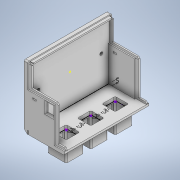
# Autodesk Inventor part: sUPORTE
Saved by Autodesk Inventor 2022 (Build 260153000, 153)
## iProperties
Created: 2022-12-13
Part Number: sUPORTE
Material: Genérico
Document SubType Name: Modeling
Designer: gugarauj07
Density: 1 g/cm^3
Appearance: Padrão
Author: gugarauj07
Autodesk Inventor part; units mm, degrees
ref_plane "YZ Plane" through (0, 0, 0) normal (1, 0, 0) x (0, 1, 0)
ref_plane "XZ Plane" through (0, 0, 0) normal (0, 1, 0) x (-1, 0, 0)
ref_plane "XY Plane" through (0, 0, 0) normal (0, 0, 1) x (1, 0, 0)
sketch "Esboço1" plane through (0, 0, 0) normal (1, 0, 0) x (0, 1, 0)
  line L0 (40.5, 60) -> (-42.5, 60)
  line L1 (-42.5, 60) -> (-42.5, -60)
  line L2 (-42.5, -60) -> (40.5, -60)
  line L3 (42.5, -58) -> (42.5, 58)
  line L4 (-42.5, 60) -> (42.5, -60) construction
  arc A0 (42.5, 58) -> (40.5, 60) centre (40.5, 58) ccw
  arc A1 (40.5, -60) -> (42.5, -58) centre (40.5, -58) ccw
  point P0 (0, 0)
  dimension "d0" = 85
  dimension "d1" = 120
  dimension "d4" = 2
  constraints: 10 end point, 4 point on circle, 4 tangent, 2 centre point, 2 parallel, 2 point on line, 1 equal radius, 1 horizontal, 1 midpoint, 1 perpendicular
  measures "d0" distance of L4.end L1.end
  measures "d1" distance of L0.end L1.end
  measures "d4" radius of A0
extrude "Extrusão1" add sketch "Esboço1" along normal blind 5
sketch "Esboço4" plane through (5, 0, 0) normal (1, 0, 0) x (0, 0, -1)
  line L0 (-60, -42.5) -> (60, -42.5) projected
  line L1 (-60, -42.5) -> (60, -42.5)
  line L2 (60, -42.5) -> (60, -47.5)
  line L3 (60, -47.5) -> (-60, -47.5)
  line L4 (-60, -47.5) -> (-60, -42.5)
  point P0 (0, 0)
  point P1 (60, -42.5)
  dimension "d33" = 5
  constraints: 8 end point, 2 parallel, 1 horizontal, 1 perpendicular
  measures "d33" distance of L1.end L2.end
extrude "Extrusão3" add sketch "Esboço4" against normal blind 5
sketch "Esboço5" plane through (5, 0, 0) normal (1, 0, 0) x (0, 0, -1)
  line L0 (-60, 40.5) -> (-60, -47.5) projected
  line L1 (60, 40.5) -> (60, -47.5) projected
  line L2 (-60, -47.5) -> (60, -47.5)
  line L3 (60, -47.5) -> (60, -42.5)
  line L4 (60, -42.5) -> (-60, -42.5)
  line L5 (-60, -42.5) -> (-60, -47.5)
  point P0 (0, 0)
  point P1 (60, -47.5)
  dimension "d36" = 5
  constraints: 8 end point, 2 parallel, 1 horizontal, 1 perpendicular, 1 point on line
  measures "d36" distance of L3.end L2.end
extrude "Extrusão4" add sketch "Esboço5" along normal blind 53.158
chamfer "Chanfro2" distance 4 angle 45 1 edges at (0, -47.5, 0)
chamfer "Chanfro3" distance 2 angle 45 1 edges at (58.158, -47.5, 0)
sketch "Esboço7" plane through (5, 0, 0) normal (1, 0, 0) x (0, 0, -1)
  circle A0 centre (-45, 0) radius 3
  circle A1 centre (45, 0) radius 3
  point P0 (0, 0)
  dimension "d61" = 6
  dimension "d62" = 6
  constraints: 2 centre point
  measures "d61" diameter of A0
  measures "d62" diameter of A1
hole "Furo3" at (5, 0, 45) direction (-1, 0, 0) diameter 4.3434 depth 16.265 tip angle 118 thread size "12-24 UNC" class "2B" standard "ANSI Unified Screw Threads"
hole "Furo4" at (5, 0, -45) direction (-1, 0, 0) diameter 4.3434 depth 16.265 tip angle 118 thread size "12-24 UNC" class "2B" standard "ANSI Unified Screw Threads"
sketch "Esboço9" plane through (4, -47.5, -60) normal (0, -1, 0) x (1, 0, 0)
  line L0 (40.5, 87.5) -> (40.5, 102.5) projected
  line L1 (23.5, 85.5) -> (38.5, 85.5) projected
  line L2 (38.5, 104.5) -> (23.5, 104.5) projected
  line L3 (21.5, 102.5) -> (21.5, 87.5) projected
  line L4 (23.5, 15.5) -> (38.5, 15.5) projected
  line L5 (43.5, 12.5) -> (31, 12.5)
  line L6 (31, 12.5) -> (16.5, 12.5)
  line L7 (16.5, 95) -> (16.5, 107.5)
  line L8 (16.5, 107.5) -> (43.5, 107.5)
  line L9 (43.5, 107.5) -> (43.5, 95)
  line L10 (38.5, 34.5) -> (23.5, 34.5) projected
  line L11 (31, 34.5) -> (31, 37.5)
  line L12 (23.5, 50.5) -> (38.5, 50.5) projected
  line L13 (31, 50.5) -> (31, 47.5)
  line L14 (38.5, 69.5) -> (23.5, 69.5) projected
  line L15 (31, 69.5) -> (31, 72.5)
  line L16 (31, 85.5) -> (31, 82.5)
  line L17 (43.5, 82.5) -> (16.5, 82.5)
  line L18 (43.5, 72.5) -> (16.5, 72.5)
  line L19 (43.5, 47.5) -> (16.5, 47.5)
  line L20 (43.5, 37.5) -> (16.5, 37.5)
  line L21 (43.5, 95) -> (43.5, 82.5)
  line L22 (16.5, 82.5) -> (16.5, 95)
  line L23 (16.5, 12.5) -> (16.5, 37.5)
  line L24 (16.5, 47.5) -> (16.5, 72.5)
  line L25 (43.5, 72.5) -> (43.5, 47.5)
  line L26 (43.5, 37.5) -> (43.5, 12.5)
  line L27 (31, 104.5) -> (31, 107.5)
  line L28 (31, 15.5) -> (31, 12.5)
  arc A0 (23.5, 104.5) -> (21.5, 102.5) centre (23.5, 102.5) ccw projected
  arc A1 (23.5, 104.5) -> (21.5, 102.5) centre (23.5, 102.5) ccw
  arc A2 (40.5, 102.5) -> (38.5, 104.5) centre (38.5, 102.5) ccw
  arc A3 (38.5, 85.5) -> (40.5, 87.5) centre (38.5, 87.5) ccw projected
  arc A4 (38.5, 85.5) -> (40.5, 87.5) centre (38.5, 87.5) ccw
  arc A5 (21.5, 87.5) -> (23.5, 85.5) centre (23.5, 87.5) ccw projected
  arc A6 (21.5, 87.5) -> (23.5, 85.5) centre (23.5, 87.5) ccw
  line L29 (21.5, 102.5) -> (21.5, 87.5)
  line L30 (23.5, 104.5) -> (31, 104.5)
  line L31 (31, 104.5) -> (38.5, 104.5)
  arc A7 (40.5, 102.5) -> (38.5, 104.5) centre (38.5, 102.5) ccw projected
  line L32 (40.5, 102.5) -> (40.5, 87.5)
  line L33 (38.5, 85.5) -> (31, 85.5)
  line L34 (23.5, 85.5) -> (31, 85.5)
  line L35 (31, 69.5) -> (29.1751, 69.5)
  arc A8 (23.5, 69.5) -> (21.5, 67.5) centre (23.5, 67.5) ccw projected
  line L36 (31, 69.5) -> (23.5, 69.5)
  line L37 (21.5, 67.5) -> (21.5, 52.5) projected
  line L38 (21.5, 67.5) -> (21.5, 52.5)
  arc A9 (21.5, 52.5) -> (23.5, 50.5) centre (23.5, 52.5) ccw projected
  line L39 (23.5, 50.5) -> (31, 50.5)
  line L40 (31, 50.5) -> (38.5, 50.5)
  arc A10 (38.5, 50.5) -> (40.5, 52.5) centre (38.5, 52.5) ccw projected
  line L41 (40.5, 52.5) -> (40.5, 67.5)
  line L42 (38.5, 69.5) -> (31, 69.5)
  line L43 (31, 34.5) -> (38.5, 34.5)
  arc A11 (40.5, 32.5) -> (38.5, 34.5) centre (38.5, 32.5) ccw projected
  arc A12 (38.5, 15.5) -> (40.5, 17.5) centre (38.5, 17.5) ccw projected
  line L44 (40.5, 32.5) -> (40.5, 17.5)
  line L45 (38.5, 15.5) -> (31, 15.5)
  arc A13 (21.5, 17.5) -> (23.5, 15.5) centre (23.5, 17.5) ccw projected
  line L46 (31, 15.5) -> (23.5, 15.5)
  line L47 (21.5, 32.5) -> (21.5, 17.5) projected
  line L48 (21.5, 17.5) -> (21.5, 32.5)
  line L49 (23.5, 34.5) -> (31, 34.5)
  arc A14 (23.5, 34.5) -> (21.5, 32.5) centre (23.5, 32.5) ccw projected
  arc A15 (23.5, 34.5) -> (21.5, 32.5) centre (23.5, 32.5) ccw
  arc A16 (21.5, 17.5) -> (23.5, 15.5) centre (23.5, 17.5) ccw
  arc A17 (38.5, 15.5) -> (40.5, 17.5) centre (38.5, 17.5) ccw
  arc A18 (40.5, 32.5) -> (38.5, 34.5) centre (38.5, 32.5) ccw
  arc A19 (38.5, 50.5) -> (40.5, 52.5) centre (38.5, 52.5) ccw
  arc A20 (21.5, 52.5) -> (23.5, 50.5) centre (23.5, 52.5) ccw
  arc A21 (23.5, 69.5) -> (21.5, 67.5) centre (23.5, 67.5) ccw
  arc A22 (40.5, 67.5) -> (38.5, 69.5) centre (38.5, 67.5) ccw projected
  arc A23 (40.5, 67.5) -> (38.5, 69.5) centre (38.5, 67.5) ccw
  point P0 (-4, 60)
  dimension "d102" = 3
  dimension "d103" = 3
  dimension "d104" = 3
  dimension "d105" = 3
  constraints: 80 end point, 25 point on circle, 21 perpendicular, 14 collinear, 12 centre point, 11 tangent, 10 vertical, 6 midpoint, 3 point on line, 2 horizontal, 1 concentric
  measures "d102" distance of L11.start L11.end
  measures "d103" distance of L13.start L13.end
  measures "d104" distance of L15.start L15.end
  measures "d105" distance of L16.start L16.end
extrude "Extrusão7" add sketch "Esboço9" along normal blind 21 contours L16 L17 L22 L7 L8 L27 L2 A0 L3 A5 L1 | L4 L28 L6 L23 L20 L11 L10 A14 L47 A13 | L12 L13 L19 L24 L18 L15 L14 A8 L37 A9
extrude "Extrusão9" add sketch "Esboço9" along normal blind 21 contours L0 A2 L2 L27 L8 L9 L21 L17 L16 L1 A3 | L4 A12 L44 A11 L10 L11 L20 L26 L5 L28 | L12 A10 L41 A22 L14 L15 L18 L25 L19 L13
fillet "Arredondamento1" radius 2 12 edges at (47.5, -58, -47.5) (20.5, -58, -47.5) (20.5, -58, -22.5) (47.5, -58, -22.5) (47.5, -58, -12.5) (20.5, -58, -12.5) (20.5, -58, 12.5) (47.5, -58, 12.5) (47.5, -58, 22.5) (20.5, -58, 22.5) (20.5, -58, 47.5) (47.5, -58, 47.5)
sketch "Esboço12" plane through (5, 0, 0) normal (1, 0, 0) x (0, 0, -1)
  line L0 (60, -42.5) -> (60, 40.5) projected
  line L1 (60, -42.5) -> (55, -42.5)
  line L2 (55, -42.5) -> (55, 7.5)
  line L3 (55, 7.5) -> (60, 7.5)
  line L4 (60, 7.5) -> (60, -42.5)
  line L5 (60, -42.5) -> (-60, -42.5) projected
  line L6 (-60, -42.5) -> (-55, -42.5)
  line L7 (-55, -42.5) -> (-55, 7.5)
  line L8 (-55, 7.5) -> (-60, 7.5)
  line L9 (-60, 7.5) -> (-60, -42.5)
  point P0 (0, 0)
  dimension "d123" = 5
  dimension "d124" = 50
  dimension "d125" = 5
  dimension "d126" = 50
  constraints: 16 end point, 4 parallel, 2 horizontal, 2 perpendicular
  measures "d123" distance of L2.end L3.end
  measures "d124" distance of L1.end L2.end
  measures "d125" distance of L8.end L7.end
  measures "d126" distance of L7.end L6.end
extrude "Extrusão10" add sketch "Esboço12" along normal blind 38
sketch "Esboço13" plane through (43, 0, 0) normal (1, 0, 0) x (0, 0, -1)
  line L0 (-60, 40.5) -> (-60, -43.5) projected
  line L1 (-60, -42.5141) -> (-58.5, -42.5141)
  line L2 (-60, -42.5141) -> (-58.5, -42.5141) construction
  line L3 (60, -42.5) -> (-60, -42.5) projected
  line L4 (-55, 7.5) -> (-60, 7.5) projected
  line L5 (-58.5, -42.5) -> (-56.5, -42.5)
  line L6 (-56.5, -42.5) -> (-56.5, 7.5)
  line L7 (-56.5, 7.5) -> (-58.5, 7.5)
  line L8 (-58.5, 7.5) -> (-58.5, -42.5)
  line L9 (58, 42.5) -> (-58, 42.5) projected
  line L10 (-57.5, 42.5) -> (-56, 42.5) construction
  line L11 (-58.5, 7.5) -> (-56.5, 7.5)
  line L12 (60, -42.5) -> (55, -42.5) projected
  line L13 (60, -42.5) -> (58.5, -42.5)
  line L14 (55, 7.5) -> (60, 7.5) projected
  line L15 (58.5, -42.5) -> (56.5, -42.5)
  line L16 (56.5, -42.5) -> (56.5, 7.5)
  line L17 (56.5, 7.5) -> (58.5, 7.5)
  line L18 (58.5, 7.5) -> (58.5, -42.5)
  point P0 (0, 0)
  dimension "d129" = 1.5
  dimension "d130" = 0
  dimension "d135" = 1.5
  dimension "d136" = 2
  constraints: 26 end point, 6 point on line, 5 horizontal, 4 parallel, 3 perpendicular, 1 collinear
  measures "d129" distance of L1.start L1.end
  measures "d130" distance between parallel lines of L1 L2
  measures "d135" distance of L3.start L13.end
  measures "d136" distance of L16.end L17.end
extrude "Extrusão11" add sketch "Esboço13" along normal blind 4 contours L4 L6 L3 L8 | L3 L16 L14 L18
extrude "Extrusão12" cut sketch "Esboço9" against normal blind 6 contours A3 L1 A5 L3 A0 L2 A2 L0 | A13 L47 A14 L10 A11 L44 A12 L4 | A9 L37 A8 L14 A22 L41 A10 L12
sketch "Esboço14" plane through (5, 0, 0) normal (1, 0, 0) x (0, 0, -1)
  line L0 (-58.5, 7.5) -> (-60, 7.5) projected
  line L1 (-58.5, 7.5) -> (-56.5, 7.5)
  line L2 (-56.5, 7.5) -> (-56.5, 41)
  line L3 (-56.5, 41) -> (-56.5, 41)
  line L4 (-58.5, 39) -> (-58.5, 7.5)
  line L5 (55, 7.5) -> (60, 7.5) projected
  line L6 (58.5055, 7.5) -> (56.5055, 7.5)
  line L7 (56.5055, 7.5) -> (56.5055, 41)
  line L8 (56.5055, 41) -> (56.5055, 41)
  line L9 (58.5055, 39) -> (58.5055, 7.5)
  line L10 (-56.5, 41) -> (56.5055, 41)
  line L11 (56.5055, 41) -> (56.5055, 39)
  line L12 (56.5055, 39) -> (-56.5, 39)
  line L13 (-56.5, 39) -> (-56.5, 41)
  arc A0 (-56.5, 41) -> (-58.5, 39) centre (-56.5, 39) ccw
  arc A1 (58.5055, 39) -> (56.5055, 41) centre (56.5055, 39) ccw
  point P0 (0, 0)
  point P1 (-58.5, 41)
  point P2 (58.5055, 41)
  dimension "d141" = 2
  dimension "d142" = 33.5
  dimension "d143" = 2
  dimension "d144" = 33.5
  dimension "d145" = 2
  dimension "d146" = 2
  dimension "d147" = 2
  constraints: 24 end point, 6 parallel, 6 point on line, 4 point on circle, 4 tangent, 3 horizontal, 3 perpendicular, 2 centre point
  measures "d141" distance of point (-58.5, 41) L2.end
  measures "d142" distance of L2.end L1.end
  measures "d143" distance of L7.end point (58.505, 41)
  measures "d144" distance of L6.end L7.end
  measures "d145" distance of L10.end L11.end
  measures "d146" radius of A0
  measures "d147" radius of A1
extrude "Extrusão13" add sketch "Esboço14" along normal blind 4
sketch "Esboço15" plane through (9, 0, 0) normal (1, 0, 0) x (0, 0, -1)
  line L0 (-56.5, 7.5) -> (-56.5, 39) projected
  line L1 (-56.5, 7.5) -> (-58.5, 7.5)
  line L2 (-58.5, 7.5) -> (-58.5, 10.5)
  line L3 (-58.5, 10.5) -> (-56.5, 10.5)
  line L4 (-56.5, 10.5) -> (-56.5, 7.5)
  line L5 (58.5, 7.5) -> (56.5, 7.5) projected
  line L6 (56.5055, 39) -> (56.5055, 7.5) projected
  line L7 (58.5, 7.5) -> (56.5055, 7.5)
  line L8 (56.5055, 7.5) -> (56.5055, 10.5)
  line L9 (56.5055, 10.5) -> (58.5, 10.5)
  line L10 (58.5, 10.5) -> (58.5, 7.5)
  point P0 (0, 0)
  dimension "d150" = 2
  dimension "d151" = 3
  dimension "d152" = 3
  constraints: 16 end point, 4 parallel, 2 horizontal, 2 perpendicular, 1 point on line
  measures "d150" distance of L2.end L3.end
  measures "d151" distance of L1.end L2.end
  measures "d152" distance of L7.end L8.end
extrude "Extrusão14" add sketch "Esboço15" along normal blind 38
sketch "Esboço16" plane through (47, 0, 0) normal (1, 0, 0) x (0, 0, -1)
  line L0 (-56.5, -42.5) -> (-58.5, -42.5) projected
  line L1 (-58.5, -42.5) -> (-58.5, 7.5) projected
  line L2 (-56.5, -42.5) -> (-58.5, -42.5)
  line L3 (-58.5, -42.5) -> (-58.5, -39.5)
  line L4 (-58.5, -39.5) -> (-56.5, -39.5)
  line L5 (-56.5, -39.5) -> (-56.5, -42.5)
  line L6 (60, -42.5) -> (58.5, -42.5) projected
  line L7 (58.5, -42.5) -> (56.5, -42.5)
  line L8 (56.5, -42.5) -> (56.5, -39.5)
  line L9 (56.5, -39.5) -> (58.5, -39.5)
  line L10 (58.5, -39.5) -> (58.5, -42.5)
  point P0 (0, 0)
  dimension "d155" = 3
  dimension "d156" = 2
  dimension "d157" = 3
  constraints: 16 end point, 4 parallel, 2 horizontal, 2 perpendicular, 1 point on line
  measures "d155" distance of L2.end L3.end
  measures "d156" distance of L8.end L9.end
  measures "d157" distance of L7.end L8.end
extrude "Extrusão15" add sketch "Esboço16" along normal blind 11
chamfer "Chanfro4" distance 2 angle 45 2 edges at (58, -39.5, 57.5) (58, -39.5, -57.5)
chamfer "Chanfro5" distance 2 angle 45 2 edges at (47, 10.5, 57.5) (47, 10.5, -57.5027)
sketch "Esboço17" plane through (9, 0, 0) normal (1, 0, 0) x (0, 0, -1)
  line L0 (-60, 42.5) -> (-57, 42.5)
  line L1 (-57, 42.5) -> (-57, 39.5)
  line L2 (-57, 39.5) -> (-60, 39.5)
  line L3 (-60, 39.5) -> (-60, 42.5)
  line L4 (60, 42.5) -> (57, 42.5)
  line L5 (57, 42.5) -> (57, 39.5)
  line L6 (57, 39.5) -> (60, 39.5)
  line L7 (60, 39.5) -> (60, 42.5)
  point P0 (0, 0)
  dimension "d166" = 3
  dimension "d167" = 3
  dimension "d168" = 3
  dimension "d169" = 3
  constraints: 16 end point, 4 parallel, 2 horizontal, 2 perpendicular
  measures "d166" distance of L1.end L2.end
  measures "d167" distance of L0.end L1.end
  measures "d168" distance of L6.end L5.end
  measures "d169" distance of L5.end L4.end
hole "Furo5" at (9, 39.5, 57) at (9, 39.5, -57) direction (-1, 0, 0) diameter 3.302 depth 12.3 tip angle 118 thread size "8-32 UNC" class "2B" standard "ANSI Unified Screw Threads"
sketch "Esboço18" plane through (4, -68.5, -60) normal (0, -1, 0) x (1, 0, 0)
  line L0 (21.5, 102.5) -> (21.5, 87.5) projected
  line L1 (21.5, 102.5) -> (21.5, 101.5)
  line L2 (21.5, 101.5) -> (19.5, 101.5)
  line L3 (19.5, 101.5) -> (19.5, 88.5)
  line L4 (19.5, 88.5) -> (21.5, 88.5)
  line L5 (21.5, 88.5) -> (21.5, 101.5)
  arc A0 (23.5, 69.5) -> (21.5, 67.5) centre (23.5, 67.5) ccw projected
  line L6 (21.5, 67.5) -> (21.5, 66.5)
  line L7 (21.5, 67.5) -> (21.5, 52.5) projected
  line L8 (21.5, 66.5) -> (19.5, 66.5)
  line L9 (19.5, 66.5) -> (19.5, 53.5)
  line L10 (19.5, 53.5) -> (21.5, 53.5)
  line L11 (21.5, 53.5) -> (21.5, 66.5)
  line L12 (21.5, 32.5) -> (21.5, 17.5) projected
  line L13 (21.5, 32.5) -> (21.5, 31.5)
  line L14 (21.5, 31.5) -> (19.5, 31.5)
  line L15 (19.5, 31.5) -> (19.5, 18.5)
  line L16 (19.5, 18.5) -> (21.5, 18.5)
  line L17 (21.5, 18.5) -> (21.5, 31.5)
  point P0 (-4, 60)
  point P1 (21.5, 18.5)
  dimension "d177" = 1
  dimension "d178" = 2
  dimension "d179" = 13
  dimension "d180" = 1
  dimension "d181" = 2
  dimension "d182" = 13
  dimension "d183" = 1
  dimension "d184" = 13
  constraints: 30 end point, 6 parallel, 3 horizontal, 3 perpendicular, 3 point on line
  measures "d177" distance of L0.start L1.end
  measures "d178" distance of L4.end L3.end
  measures "d179" distance of L3.end L2.end
  measures "d180" distance of L6.start L6.end
  measures "d181" distance of L10.end L9.end
  measures "d182" distance of L9.end L8.end
  measures "d183" distance of L12.start L13.end
  measures "d184" distance of L15.end L14.end
extrude "Extrusão16" cut sketch "Esboço18" against normal blind 19
sketch "Esboço20" plane through (0, 40.5, 60) normal (0, 0, 1) x (1, 0, 0)
  line L0 (43, -33) -> (43, -83) projected
  line L1 (43, -33) -> (42, -33)
  line L2 (42, -33) -> (42, -34)
  line L3 (42, -34) -> (43, -34)
  line L4 (43, -34) -> (43, -33)
  line L5 (42, -34) -> (29, -34)
  line L6 (29, -34) -> (29, -51)
  line L7 (29, -51) -> (42, -51)
  line L8 (42, -51) -> (42, -34)
  point P0 (0, -40.5)
  dimension "d187" = 1
  dimension "d188" = 1
  dimension "d189" = 13
  dimension "d190" = 17
  constraints: 16 end point, 4 parallel, 2 horizontal, 2 perpendicular
  measures "d187" distance of L3.end L2.end
  measures "d188" distance of L2.end L1.end
  measures "d189" distance of L7.end L6.end
  measures "d190" distance of L6.end L5.end
extrude "Extrusão17" cut sketch "Esboço20" against normal blind 5 contours L8 L7 L6 L5
sketch "Esboço21" plane through (0, 40.5, 60) normal (0, 0, 1) x (1, 0, 0)
  line L0 (12, -41.0317) -> (17, -41.0317)
  line L1 (17, -41.0317) -> (17, -39.0317)
  line L2 (17, -39.0317) -> (12, -39.0317)
  line L3 (12, -39.0317) -> (12, -41.0317)
  point P0 (0, -40.5)
  dimension "d195" = 5
  dimension "d196" = 2
  constraints: 8 end point, 2 parallel, 1 horizontal, 1 perpendicular
  measures "d195" distance of L2.end L1.end
  measures "d196" distance of L1.end L0.end
extrude "Extrusão18" cut sketch "Esboço21" against normal through all
